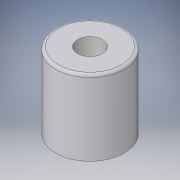
# Autodesk Inventor part: Part4
Saved by Autodesk Inventor 2016 (Build 200138000, 138)
## iProperties
Created: 2015-12-15
Part Number: Part4
Material: ABS Plastic
Document SubType Name: Modeling
Designer: Nanjar
Density: 1.06 g/cm^3
Appearance: Smooth - White
Author: Nanjar
Autodesk Inventor part; units mm, degrees
ref_plane "YZ Plane" through (0, 0, 0) normal (1, 0, 0) x (0, 1, 0)
ref_plane "XZ Plane" through (0, 0, 0) normal (0, 1, 0) x (-1, 0, 0)
ref_plane "XY Plane" through (0, 0, 0) normal (0, 0, 1) x (1, 0, 0)
sketch "Sketch1" plane through (0, 0, 0) normal (0, 1, 0) x (-1, 0, 0)
  circle A0 centre (0, 0) radius 2.5
  dimension "d0" = 5
  constraints: 1 centre point, 1 coincident
  measures "d0" diameter of A0
extrude "Extrusion1" add sketch "Sketch1" along normal blind 5.5
fillet "Fillet1" radius 0.2 1 edges at (2.5, 5.5, 0)
sketch "Sketch2" plane through (0, 5.5, 0) normal (0, 1, 0) x (1, 0, 0)
  circle A0 centre (0, 0) radius 0.9
  dimension "d4" = 1.8
  constraints: 1 centre point, 1 coincident
  measures "d4" diameter of A0
extrude "Extrusion2" cut sketch "Sketch2" against normal blind 6
body "Solid1"
